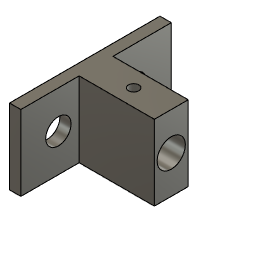
Rail_Attachment_Poll v6 (Autodesk Fusion 360 design; units mm, degrees)
Autodesk Fusion 360 part; units mm, degrees
note: some values were not read from the file. Set by a fixed rule: which sketch regions a step uses.
sketch "Sketch1" plane through (0, 0, 0) normal (0, 0, 1) x (1, 0, 0)
  line L0 (0, 0) -> (0, 20)
  line L1 (0, 20) -> (3, 20)
  line L2 (0, 0) -> (3, 0)
  line L3 (3, 0) -> (3, 20)
  dimension "d1" = 20
  constraint coincident L0.start L2.start
  constraint vertical L0
  constraint perpendicular L0 L1
  constraint horizontal L2
  constraint perpendicular L1 L3
  measures "d1" distance of L0.start L0.end
extrude "Extrude1" add sketch "Sketch1" along normal blind 60
sketch "Sketch2" plane through (3, 0, 0) normal (1, 0, 0) x (0, 0, -1)
  line L0 (0, 0) -> (0, 20)
  line L1 (0, 20) -> (-60, 20)
  line L2 (-60, 20) -> (-60, 0)
  line L3 (-60, 0) -> (0, 0)
  line L4 (-60, 10) -> (-40, 10)
  line L5 (0, 10) -> (-20, 10)
  circle A0 centre (-10, 10) radius 3.125
  circle A1 centre (-50, 10) radius 3.125
  dimension "d5" = 20
  dimension "d6" = 20
  dimension "d7" = 6.25
  dimension "d8" = 6.25
  constraint midpoint L2 L4.start
  constraint perpendicular L2 L4
  constraint midpoint L0 L5.start
  constraint perpendicular L0 L5
  constraint midpoint L5 A0.centre
  constraint midpoint L4 A1.centre
  measures "d5" distance of L4.start L4.end
  measures "d6" distance of L5.start L5.end
  measures "d7" diameter of A0
  measures "d8" diameter of A1
extrude "Extrude2" cut sketch "Sketch2" against normal blind 18 contours L4 A1 | L4 A1 | L5 A0 | L5 A0
sketch "Sketch3" plane through (3, 0, 0) normal (1, 0, 0) x (0, 0, -1)
  circle A0 centre (-50, 10) radius 3.125
  circle A1 centre (-10, 10) radius 3.125
  line L0 (0, 0) -> (0, 20)
  line L1 (0, 20) -> (-60, 20)
  line L2 (-60, 20) -> (-60, 0)
  line L3 (-60, 0) -> (0, 0)
  line L4 (-30, 20) -> (-30, 0)
  circle A2 centre (-30, 10) radius 10
  circle A3 centre (-30, 10) radius 5.25
  circle A4 centre (-30, 10) radius 7.25
  dimension "d11" = 10.5
  dimension "d13" = 14.5
  constraint midpoint L1 L4.start
  constraint midpoint L3 L4.end
  constraint midpoint L4 A2.centre
  constraint coincident L4.start A2
  constraint concentric A2 A3
  constraint concentric A2 A4
  measures "d11" diameter of A3
  measures "d13" diameter of A4
extrude "Extrude3" add sketch "Sketch3" along normal blind 20 contours L4 A3 A4 | L4 A3 A4
sketch "Sketch4" plane through (0, 20, 0) normal (0, 1, 0) x (-1, 0, 0)
  line L0 (-3, 0) -> (0, 0)
  line L1 (0, 0) -> (0, 60)
  line L2 (0, 60) -> (-3, 60)
  line L3 (-3, 60) -> (-3, 0)
  line L4 (-3, 30) -> (-23, 30)
  circle A0 centre (-13, 30) radius 1.375
  dimension "d16" = 2.75
  constraint midpoint L3 L4.start
  constraint perpendicular L3 L4
  constraint midpoint L4 A0.centre
  measures "d16" diameter of A0
extrude "Extrude4" cut sketch "Sketch4" against normal blind 41 contours L4 A0 | L4 A0
extrude "Extrude5" add 1 faces at (3, 7.9628, 30.875) along direction (1, 0, 0) blind 2
delete_face "DeleteFace1" 1 faces at (2, 10.3111, 6.8905)
delete_face "DeleteFace2" 1 faces at (2, 10.3111, 46.8905)
sketch "Sketch5" plane through (0, 0, 0) normal (-1, 0, 0) x (0, 0, 1)
  line L0 (0, 20) -> (0, 0)
  line L1 (0, 0) -> (60, 0)
  line L2 (60, 0) -> (60, 20)
  line L3 (60, 20) -> (0, 20)
  line L4 (30, 20) -> (30, 0)
  line L5 (30, 10) -> (50, 10)
  circle A0 centre (40, 10) radius 3.375
  line L6 (30, 10) -> (20, 10)
  circle A1 centre (20, 10) radius 3.375
  dimension "d21" = 20
  dimension "d24" = 6.75
  dimension "d25" = 10
  dimension "d26" = 6.75
  constraint midpoint L3 L4.start
  constraint midpoint L1 L4.end
  constraint midpoint L4 L5.start
  constraint perpendicular L4 L5
  constraint midpoint L5 A0.centre
  constraint perpendicular L4 L6
  constraint coincident L6.end A1.centre
  measures "d21" distance of L5.start L5.end
  measures "d24" diameter of A0
  measures "d25" distance of L5.start L6.end
  measures "d26" diameter of A1
extrude "Extrude6" cut sketch "Sketch5" against normal blind 4 contours L5 A0 | L5 A0 | A1
sketch "Sketch6" plane through (23, 0, 0) normal (1, 0, 0) x (0, 0, -1)
  circle A0 centre (-30, 10) radius 5.25
  circle A1 centre (-30, 10) radius 7.25
  circle A2 centre (-30, 10) radius 3.75
  circle A3 centre (-30, 10) radius 5
  dimension "d29" = 7.5
  dimension "d30" = 10
  constraint concentric A0 A2
  constraint concentric A0 A3
  measures "d29" diameter of A2
  measures "d30" diameter of A3
extrude "Extrude7" add sketch "Sketch6" against normal blind 21 contours A3
sketch "Sketch7" plane through (0, 20, 0) normal (0, 1, 0) x (-1, 0, 0)
  line L0 (-3, 0) -> (0, 0)
  line L1 (0, 0) -> (0, 60)
  line L2 (0, 60) -> (-3, 60)
  line L3 (-3, 60) -> (-3, 0)
  line L4 (-3, 30) -> (-23, 30)
  circle A0 centre (-13, 30) radius 1.375
  dimension "d33" = 2.75
  constraint midpoint L3 L4.start
  constraint perpendicular L3 L4
  constraint midpoint L4 A0.centre
  measures "d33" diameter of A0
extrude "Extrude8" cut sketch "Sketch7" against normal blind 23 contours L4 A0 | L4 A0
extrude "Extrude9" cut 1 faces at (23, 10.621, 23.4632) along direction (-1, 0, 0) blind 20
extrude "Extrude10" cut 1 faces at (5, 13.8616, 33.4131) along direction (-1, 0, 0) blind 2
sketch "Sketch8" plane through (3, 0, 0) normal (1, 0, 0) x (0, 0, -1)
  circle A0 centre (-30, 10) radius 5
  circle A1 centre (-40, 10) radius 3.375
  circle A2 centre (-20, 10) radius 3.375
  line L0 (0, 0) -> (0, 20)
  line L1 (0, 20) -> (-60, 20)
  line L2 (-60, 20) -> (-60, 0)
  line L3 (-60, 0) -> (0, 0)
  line L4 (-20, 10) -> (-10, 10)
  line L5 (-40, 10) -> (-50, 10)
  line L6 (-50, 10) -> (-50, 20)
  line L7 (-50, 0) -> (-50, 1)
  line L8 (-50, 1) -> (-50, 10)
  line L9 (-10, 10) -> (-10, 20)
  line L10 (-10, 10) -> (-10, 0)
  constraint coincident A2.centre L4.start
  constraint horizontal L4
  constraint coincident A1.centre L5.start
  constraint horizontal L5
  constraint coincident L1 L6.end
  constraint perpendicular L1 L6
  constraint coincident L3 L7.start
  constraint perpendicular L3 L7
  constraint perpendicular L5 L8
  constraint coincident L1 L9.end
  constraint perpendicular L1 L9
  constraint coincident L3 L10.end
  constraint perpendicular L3 L10
extrude "Extrude11" cut sketch "Sketch8" against normal blind 22 contours L0 L1 L3 L9 L10 | L1 L2 L3 L6 L7 L8
sketch "Sketch9" plane through (23, 0, 0) normal (1, 0, 0) x (0, 0, -1)
  circle A0 centre (-30, 10) radius 3.75
  circle A1 centre (-30, 10) radius 5
  circle A2 centre (-30, 10) radius 4.5
  dimension "d42" = 9
  constraint concentric A0 A2
  measures "d42" diameter of A2
extrude "Extrude12" cut sketch "Sketch9" against normal blind 20 contours A1
sketch "Sketch10" plane through (3, 0, 0) normal (1, 0, 0) x (0, 0, -1)
  circle A0 centre (-30, 10) radius 4.5
  line L0 (-50, 20) -> (-50, 0)
  line L1 (-50, 0) -> (-10, 0)
  line L2 (-10, 0) -> (-10, 20)
  line L3 (-10, 20) -> (-50, 20)
  circle A1 centre (-40, 10) radius 3.375
  circle A2 centre (-20, 10) radius 3.375
  line L4 (-30, 10) -> (-34.5, 10)
  line L5 (-34.5, 10) -> (-34.5, 20)
  line L6 (-30, 10) -> (-25.5, 10)
  line L7 (-25.5, 10) -> (-25.5, 10.6291)
  line L8 (-25.5, 10.6291) -> (-25.5, 20)
  line L9 (-34.5, 10) -> (-34.5, 0)
  line L10 (-25.5, 10) -> (-25.5, 0)
  constraint coincident A0.centre L4.start
  constraint coincident A0 L4.end
  constraint horizontal L4
  constraint coincident L3 L5.end
  constraint tangent A0 L5
  constraint coincident A0 L6.end
  constraint perpendicular L5 L6
  constraint tangent A0 L7
  constraint coincident L3 L8.end
  constraint perpendicular L3 L8
  constraint coincident L1 L9.end
  constraint tangent A0 L9
  constraint coincident L1 L10.end
  constraint tangent A0 L10
fillet "Fillet1" radius 5.5 1 edges at (3, 8.3727, 34.1955)
extrude "Extrude13" cut sketch "Sketch10" along normal blind 9 contours L1 L2 L3 L7 L8 L10 | L0 L1 L3 L5 L9
sketch "Sketch11" plane through (3, 0, 0) normal (1, 0, 0) x (0, 0, -1)
  arc A0 (-30, 20) -> (-34.5, 18.9303) centre (-30, 10) ccw
  line L0 (-30, 20) -> (-50, 20)
  line L1 (-50, 20) -> (-50, 0)
  line L2 (-50, 0) -> (-30, 0)
  arc A1 (-34.5, 1.0697) -> (-30, 0) centre (-30, 10) ccw
  line L3 (-34.5, 1.0697) -> (-34.5, 18.9303)
  circle A2 centre (-40, 10) radius 3.375
  line L4 (-34.5, 10) -> (-34.5, 20)
  line L5 (-34.5, 10) -> (-25.5, 10)
  line L6 (-25.5, 10) -> (-25.5, 20)
  line L7 (-25.5, 20) -> (-34.5, 20)
  line L8 (-34.5, 20) -> (-34.5, 0)
  line L9 (-34.5, 0) -> (-25.5, 0)
  line L10 (-25.5, 0) -> (-25.5, 10)
  circle A3 centre (-30, 10) radius 4.5
  constraint midpoint L3 L4.start
  constraint coincident L0 L4.end
  constraint perpendicular L0 L4
  constraint perpendicular L3 L5
  constraint perpendicular L5 L6
  constraint perpendicular L4 L7
  constraint coincident L2 L8.end
  constraint perpendicular L2 L8
  constraint perpendicular L8 L9
  constraint perpendicular L5 L10
  constraint concentric A0 A3
  constraint coincident L4.start A3
extrude "Extrude14" add sketch "Sketch11" along normal blind 20 contours A0 L3 L4 L6 L7 L8 A3 | A0 L0 L4 L7 L8 | A1 L3 L8 L9 L10 A3 | L2 A1 L8 L9
sketch "Sketch12" plane through (0, 20, 0) normal (0, 1, 0) x (-1, 0, 0)
  line L0 (0, 50) -> (-3, 50)
  line L1 (-3, 50) -> (-3, 34.5)
  line L2 (-3, 34.5) -> (-23, 34.5)
  line L3 (-23, 34.5) -> (-23, 25.5)
  line L4 (-23, 25.5) -> (-3, 25.5)
  line L5 (-3, 25.5) -> (-3, 10)
  line L6 (-3, 10) -> (0, 10)
  line L7 (0, 10) -> (0, 50)
  line L8 (-23, 30) -> (-3, 30)
  circle A0 centre (-13, 30) radius 1.375
  dimension "d51" = 2.75
  constraint midpoint L3 L8.start
  constraint perpendicular L5 L8
  constraint midpoint L8 A0.centre
  measures "d51" diameter of A0
extrude "Extrude15" cut sketch "Sketch12" against normal blind 25 contours L8 A0 | L8 A0
